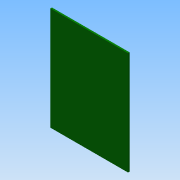
# Autodesk Inventor part: MainPCB
Saved by Autodesk Inventor 2014 (Build 180170000, 170)
## iProperties
Created: 2014-01-06
Part Number: MainPCB
Material: Silicon Nitride
Document SubType Name: Modeling
Designer: davidgitz
Density: 3.18 g/cm^3
Appearance: Dark Green
Author: davidgitz
Autodesk Inventor part; units mm, degrees
ref_plane "YZ Plane" through (0, 0, 0) normal (1, 0, 0) x (0, 1, 0)
ref_plane "XZ Plane" through (0, 0, 0) normal (0, 1, 0) x (-1, 0, 0)
ref_plane "XY Plane" through (0, 0, 0) normal (0, 0, 1) x (1, 0, 0)
sketch "Sketch1" plane through (0, 0, 0) normal (0, 0, 1) x (1, 0, 0)
  line L0 (7.6734, 93.6724) -> (-119.3266, 93.6724)
  line L1 (-119.3266, 93.6724) -> (-119.3266, -78.2856)
  line L2 (-119.3266, -78.2856) -> (7.6734, -78.2856)
  line L3 (7.6734, -78.2856) -> (7.6734, 93.6724)
  circle A0 centre (-4.417, -116.6396) radius 1.5875 projected
  circle A1 centre (-4.417, -166.9316) radius 1.5875 projected
  circle A2 centre (-106.6266, -166.9316) radius 1.5875 projected
  circle A3 centre (-106.6266, -116.6396) radius 1.5875 projected
  arc A4 (-154.2516, -90.9856) -> (-163.7766, -100.5106) centre (-154.2516, -100.5106) ccw projected
  line L4 (-163.7766, -180.5206) -> (-163.7766, -100.5106) projected
  arc A5 (-163.7766, -180.5206) -> (-154.2516, -190.0456) centre (-154.2516, -180.5206) ccw projected
  line L5 (42.5984, -190.0456) -> (-154.2516, -190.0456) projected
  arc A6 (42.5984, -190.0456) -> (52.1234, -180.5206) centre (42.5984, -180.5206) ccw projected
  line L6 (52.1234, -100.5106) -> (52.1234, -180.5206) projected
  arc A7 (52.1234, -100.5106) -> (42.5984, -90.9856) centre (42.5984, -100.5106) ccw projected
  line L7 (-154.2516, -90.9856) -> (42.5984, -90.9856) projected
  line L8 (7.6734, 106.3724) -> (7.6734, -198.4276) projected
  line L9 (-119.3266, 106.3724) -> (-119.3266, -198.4276) projected
  line L10 (-93.9266, 106.3724) -> (-119.3266, 106.3724) projected
  point P0 (0, 0)
  dimension "d1" = 12.7
  dimension "d4" = 12.7
  constraints: 8 end point, 2 parallel, 2 point on line, 1 horizontal, 1 perpendicular
  measures "d1" distance between parallel lines of L2 L7
  measures "d4" distance between parallel lines of L10 L0
extrude "Extrusion1" add sketch "Sketch1" along normal blind 2.54 contours L3 L2 L1 L0
body "Solid1"
